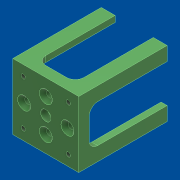
# Autodesk Inventor part: 901-4250 house
Saved by Autodesk Inventor 2018 (Build 220112000, 112)
## iProperties
Created: 2019-12-10
Part Number: 901-4250 house
Material: Generic
Document SubType Name: Modeling
Designer: Bunny320
Density: 1 g/cm^3
Appearance: Smooth - Dark Forest Green
Author: Bunny320
Autodesk Inventor part; units mm, degrees
ref_plane "YZ Plane" through (0, 0, 0) normal (1, 0, 0) x (0, 1, 0)
ref_plane "XZ Plane" through (0, 0, 0) normal (0, 1, 0) x (-1, 0, 0)
ref_plane "XY Plane" through (0, 0, 0) normal (0, 0, 1) x (1, 0, 0)
sketch "Sketch1" plane through (0, 0, 0) normal (0, 1, 0) x (-1, 0, 0)
  line L0 (-19, 19) -> (19, 19)
  line L1 (19, 19) -> (19, -19)
  line L2 (19, -19) -> (-19, -19)
  line L3 (-19, -19) -> (-19, 19)
  line L4 (-19, 19) -> (19, -19) construction
  line L5 (19, 19) -> (-19, -19) construction
  point P0 (0, 0)
  dimension "d0" = 38
  constraints: 12 end point, 2 midpoint, 2 parallel, 2 perpendicular, 1 horizontal
  measures "d0" distance of L0.start L0.end
extrude "Extrusion1" add sketch "Sketch1" along normal blind 6
sketch "Sketch2" plane through (0, 6, 0) normal (0, 1, 0) x (1, 0, 0)
  line L0 (19, 19) -> (-19, 19) projected
  line L1 (-19, 19) -> (-11, 19)
  line L2 (-11, 19) -> (-11, 15.4919)
  line L3 (-15.4919, 11) -> (-19, 11)
  line L4 (-19, 11) -> (-19, 19)
  circle A0 centre (0, 0) radius 19
  dimension "d3" = 38
  dimension "d5" = 8
  constraints: 8 end point, 2 parallel, 2 perpendicular, 2 point on circle, 1 centre point, 1 coincident, 1 horizontal
  measures "d3" diameter of A0
  measures "d5" distance between parallel lines of L4 L2
extrude "Extrusion2" add sketch "Sketch2" along normal blind 45 contours L2 A0 L3 L4 L0
sketch "Sketch3" plane through (0, 0, 0) normal (0, 1, 0) x (-1, 0, 0)
  line L0 (0, -26.6) -> (0, 26.6) projected
  line L1 (-26.6, 0) -> (26.6, 0) projected
  point P0 (0, -9.5)
  point P1 (0, 9.5)
  point P2 (-12.5, 0)
  point P3 (12.5, 0)
  dimension "d48" = 19
  dimension "d49" = 25
  dimension "d50" = 9.5
  dimension "d51" = 12.5
  constraints: 4 point on line
  measures "d48" distance of point (0, 9.5) point (0, -9.5)
  measures "d49" distance of point (-12.5, 0) point (12.5, 0)
  measures "d50" distance from line of L1 point (0, -9.5)
  measures "d51" distance from line of L0 point (12.5, 0)
hole "Hole1" at (0, 0, -9.5) at (12.5, 0, 0) at (0, 0, 9.5) at (-12.5, 0, 0) direction (0, 1, 0) diameter 3.4 end through all countersink diameter 7.5 countersink angle 90 clearance for "Countersunk Flat Head Hex Socket Screw DIN EN ISO 10642" size "M3" standard "DIN"
fillet "Fillet1" radius 5 2 edges at (-11, 6, -17.246) (-17.246, 6, -11)
fillet "Fillet1" radius 2 1 edges at (-13.435, 6, -13.435)
sketch "Sketch5" plane through (0, 51, 0) normal (0, 1, 0) x (1, 0, 0)
  point P0 (0, 0)
  point P1 (-15.5, 15.5)
  dimension "d27" = 15.5
  dimension "d28" = 15.5
  measures "d27" horizontal distance of point (0, 0) point (-15.5, 15.5)
  measures "d28" horizontal distance of point (0, 0) point (-15.5, 15.5)
hole "Hole3" at (-15.5, 51, -15.5) direction (0, -1, 0) diameter 2.459 depth 20 tip angle 118 thread size "M3x0.5" class "6H" standard "ISO Metric profile"
sketch "Sketch4" plane through (0, 0, 0) normal (0, 1, 0) x (-1, 0, 0)
  line L0 (-13, 13) -> (13, 13)
  line L1 (13, 13) -> (13, -13)
  line L2 (13, -13) -> (-13, -13)
  line L3 (-13, -13) -> (-13, 13)
  line L4 (-13, 13) -> (13, -13) construction
  line L5 (13, 13) -> (-13, -13) construction
  point P0 (0, 0)
  dimension "d19" = 26
  constraints: 12 end point, 2 midpoint, 2 parallel, 2 perpendicular, 1 coincident, 1 horizontal
  measures "d19" distance of L0.start L0.end
hole "Hole2" at (-13, 0, -13) direction (0, 1, 0) diameter 2.459 depth 15 tip angle 118 thread size "M3x0.5" class "6H" standard "ISO Metric profile"
pattern_circular "Circular Pattern1" count 4 over 360 about axis through (0, -10, 0) along (0, 1, 0) of "Extrusion2", "Hole2", "Hole3", "Fillet1"
sketch "Sketch6" plane through (0, 6, 0) normal (0, 1, 0) x (1, 0, 0)
  point P0 (0, 0)
  point P1 (0, 0)
  constraints: 1 coincident
hole "Hole4" at (0, 6, 0) direction (0, -1, 0) diameter 6 end through all counterbore diameter 12 counterbore depth 2
equation "\"d50\" = 0.5 * d48"
equation "\"d51\" = 0.5 * d49"
equation "\"d28\" = d27"
body "Solid1"
